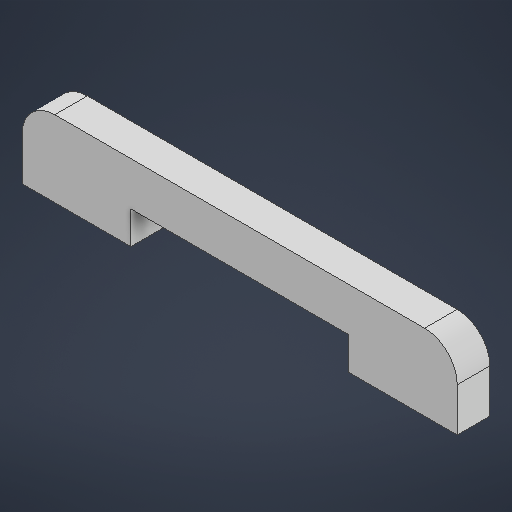
# Autodesk Inventor part: Stopper
Saved by Autodesk Inventor 2027 (Build 310192000, 192)
## iProperties
Created: 2026-06-01
Part Number: Stopper
Material: Generic
Document SubType Name: Modeling
Designer: alexy
Density: 1 g/cm^3
Appearance: Default
Author: alexy
Autodesk Inventor part; units mm, degrees
ref_plane "YZ Plane" through (0, 0, 0) normal (1, 0, 0) x (0, 1, 0)
ref_plane "XZ Plane" through (0, 0, 0) normal (0, 1, 0) x (-1, 0, 0)
ref_plane "XY Plane" through (0, 0, 0) normal (0, 0, 1) x (1, 0, 0)
sketch "Sketch1" plane through (0, 0, 0) normal (0, 0, 1) x (1, 0, 0)
  line L0 (0, 0) -> (0, 7)
  line L1 (0, 7) -> (40, 7)
  line L2 (40, 7) -> (40, 0)
  line L3 (40, 0) -> (30, 0)
  line L4 (30, 0) -> (30, 3)
  line L5 (30, 3) -> (10, 3)
  line L6 (10, 3) -> (10, 0)
  line L7 (10, 0) -> (0, 0)
  dimension "d0" = 40
  dimension "d1" = 10
  dimension "d2" = 10
  dimension "d3" = 3
  dimension "d4" = 7
  constraints: 16 end point, 7 perpendicular, 1 point on line, 1 vertical
  measures "d0" distance of L0.end L1.end
  measures "d1" distance of L2.end L3.end
  measures "d2" distance of L6.end L0.start
  measures "d3" distance from line of L3.end L5
  measures "d4" distance of L0.start L0.end
extrude "Extrusion1" add sketch "Sketch1" along normal blind 3
fillet "Fillet1" radius 3 2 edges at (40, 7, 1.5) (0, 7, 1.5)
body "Solid1"
